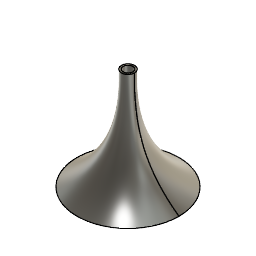
Speaker (Autodesk Fusion 360 design; units mm, degrees)
part number: 2026-02-14-14-06-01-764
Autodesk Fusion 360 part; units mm, degrees
sketch "Sketch1" plane through (0, 0, 0) normal (0, 0, 1) x (1, 0, 0)
  line L0 (0, 0) -> (400, 0)
  line L1 (400, 0) -> (400, 170)
  line L2 (400, 170) -> (0, 170)
  line L3 (0, 170) -> (0, 0)
  line L4 (0, 170) -> (80, 170)
  line L5 (0, 0) -> (8, 0)
  spline S0 degree 5 poles (80, 170) (76.8152, 167.7798) (70.6015, 163.2341) (61.7483, 156.0994) (50.8944, 145.9439) (39.0153, 132.108) (28.9632, 117.0366) (20.8682, 100.6418) (14.7663, 82.8992) (10.5427, 63.8866) (8.0398, 43.7104) (7.2935, 26.7201) (7.3941, 13.5309) (7.7499, 4.5428) (8, 0) knots 0 0 0 0 0 0 0.1 0.2 0.3 0.4 0.5 0.6 0.7 0.8 0.9 1 1 1 1 1 1
  spline S1 degree 5 poles (85, 170) (81.8462, 167.7755) (75.6881, 163.2214) (66.8996, 156.0753) (56.0935, 145.9067) (44.206, 132.0582) (34.0715, 116.9786) (25.8147, 100.5803) (19.4693, 82.8397) (14.9247, 63.8344) (12.0297, 43.6706) (10.9177, 26.6941) (10.7167, 13.5171) (10.8594, 4.5381) (11, 0) knots 0 0 0 0 0 0 0.1 0.2 0.3 0.4 0.5 0.6 0.7 0.8 0.9 1 1 1 1 1 1
  spline S2 degree 5 poles (87, 170) (83.8462, 167.7755) (77.6881, 163.2214) (68.8996, 156.0753) (58.0935, 145.9067) (46.206, 132.0582) (36.0715, 116.9786) (27.8147, 100.5803) (21.4693, 82.8397) (16.9247, 63.8344) (14.0297, 43.6706) (12.9177, 26.6941) (12.7167, 13.5171) (12.8594, 4.5381) (13, 0) knots 0 0 0 0 0 0 0.1 0.2 0.3 0.4 0.5 0.6 0.7 0.8 0.9 1 1 1 1 1 1
  point P0 (23.1219, 104.3533)
  point P1 (28.1219, 104.3533)
  point P2 (30.1219, 104.3533)
  dimension "d1" = 400
  dimension "d2" = 170
  dimension "d3" = 80
  dimension "d4" = 8
  constraint horizontal L0
  constraint vertical L1
  constraint horizontal L2
  constraint vertical L3
  constraint coincident L0.start L3.end
  constraint perpendicular L3 L4
  constraint perpendicular L3 L5
  constraint coincident L0 S1.end
  constraint coincident L0 S2.end
  measures "d1" distance of L0.start L0.end
  measures "d2" distance of L0.start L2.end
  measures "d3" distance of L2.end L4.end
  measures "d4" distance of L0.start L5.end
revolve "Revolve1" add sketch "Sketch1" angle 360 about axis through (0, 170, 0) along (0, -1, 0) contours L0 L2 L3 L4 L5 S0 | L0 L2 S0 S1
revolve "Revolve2" cut sketch "Sketch1" angle 360 about axis through (0, 170, 0) along (0, -1, 0) contours L0 L2 L3 L4 L5 S0
move_body "Move1" bodies 1 to x (1, 0, 0) y (0, 0, -1) z (0, 1, 0) at (0, 85, 185)
move_body "Move2" bodies 1 to x (1, 0, 0) y (0, 1, 0) z (0, 0, 1) at (0, 0, -15)
